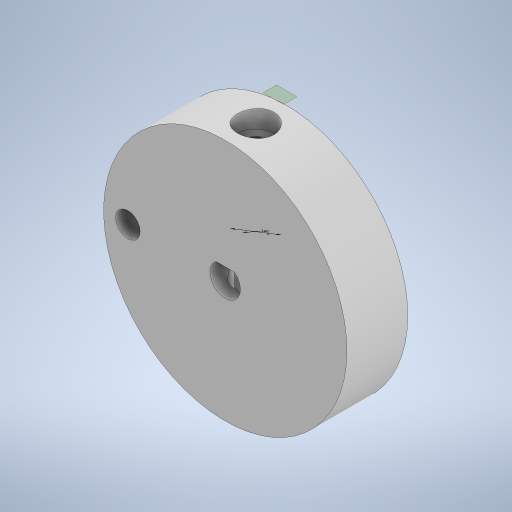
# Autodesk Inventor part: crank
Saved by Autodesk Inventor 2024 (Build 280153000, 153)
## iProperties
Created: 2024-03-27
Part Number: crank
Material: 一般
Document SubType Name: Modeling
Designer: user
Density: 1 g/cm^3
Appearance: 預設
Author: user
Autodesk Inventor part; units mm, degrees
ref_plane "YZ Plane" through (0, 0, 0) normal (1, 0, 0) x (0, 1, 0)
ref_plane "XZ Plane" through (0, 0, 0) normal (0, 1, 0) x (-1, 0, 0)
ref_plane "XY Plane" through (0, 0, 0) normal (0, 0, 1) x (1, 0, 0)
sketch "草圖1" plane through (0, 0, 0) normal (0, 0, 1) x (1, 0, 0)
  arc A0 (-1.5263, 1.98) -> (1.5263, 1.98) centre (0, 0) ccw
  line L0 (1.5263, 1.98) -> (-1.5263, 1.98)
  circle A1 centre (0, 0) radius 20
  point P0 (0, -2.5)
  dimension "d0" = 5
  dimension "d2" = 4.48
  dimension "d3" = 40
  constraints: 3 point on circle, 2 centre point, 2 coincident, 2 end point
  measures "d0" diameter of A0
  measures "d2" distance from line of point (0, -2.5) L0
  measures "d3" diameter of A1
extrude "擠出1" add sketch "草圖1" along normal blind 10
sketch "草圖2" plane through (-1.5263, 1.98, 0) normal (0, -1, 0) x (1, 0, 0)
  line L0 (3.2584, 8) -> (4.9904, 5)
  line L1 (4.9904, 5) -> (3.2584, 2)
  line L2 (3.2584, 2) -> (-0.2057, 2)
  line L3 (-0.2057, 2) -> (-1.9378, 5)
  line L4 (-1.9378, 5) -> (-0.2057, 8)
  line L5 (-0.2057, 8) -> (3.2584, 8)
  point P0 (1.5263, 0)
  point P1 (1.5263, 5)
  point P2 (1.5263, 8)
  constraints: 12 end point, 1 midpoint, 13 other
extrude "擠出2" cut sketch "草圖2" against normal blind 2.5
extrude "擠出3" cut sketch "草圖2" along normal through all
sketch "草圖4" plane through (-1.5263, 4.48, 0) normal (0, -1, 0) x (1, 0, 0)
  circle A0 centre (1.5263, 5) radius 1.5
  circle A1 centre (1.5263, 5) radius 3
  point P0 (1.5263, 0)
  dimension "d11" = 3
  dimension "d12" = 6
  constraints: 2 centre point, 1 coincident
  measures "d11" diameter of A0
  measures "d12" diameter of A1
extrude "擠出4" cut sketch "草圖4" against normal through all contours A0
ref_plane "工作平面1" through (-1.5263, 21.98, 0) normal (0, -1, 0) x (1, 0, 0)
sketch "草圖5" plane through (-1.5263, 21.98, 0) normal (0, -1, 0) x (1, 0, 0)
  circle A0 centre (1.5263, 5) radius 1.5 projected
  circle A1 centre (1.5263, 5) radius 3
  point P0 (1.5263, 0)
  dimension "d16" = 6
  constraints: 1 centre point, 1 coincident
  measures "d16" diameter of A1
extrude "擠出5" cut sketch "草圖5" along normal blind 5 contours A0 | A1
sketch "草圖6" plane through (0, 0, 0) normal (0, 0, -1) x (-1, 0, 0)
  circle A0 centre (16, 0) radius 2
  point P0 (0, 0)
  dimension "d19" = 4
  dimension "d20" = 16
  constraints: 1 centre point
  measures "d19" diameter of A0
  measures "d20" distance of point (0, 0) A0.centre
extrude "擠出6" cut sketch "草圖6" against normal through all
